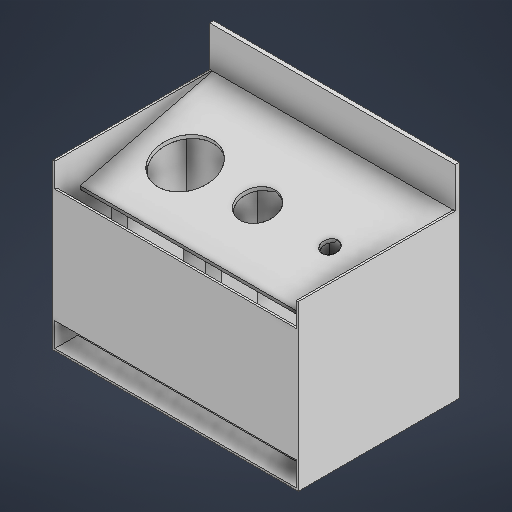
# Autodesk Inventor part: collectingbox
Saved by Autodesk Inventor 2026.2 (Build 302298000, 298)
## iProperties
Created: 2026-03-08
Part Number: collectingbox
Material: Generic
Document SubType Name: Modeling
Designer: danda
Density: 1 g/cm^3
Appearance: Default
Author: danda
Autodesk Inventor part; units mm, degrees
ref_plane "YZ Plane" through (0, 0, 0) normal (1, 0, 0) x (0, 1, 0)
ref_plane "XZ Plane" through (0, 0, 0) normal (0, 1, 0) x (-1, 0, 0)
ref_plane "XY Plane" through (0, 0, 0) normal (0, 0, 1) x (1, 0, 0)
sketch "Sketch1" plane through (0, 0, 0) normal (0, 0, 1) x (1, 0, 0)
  line L0 (-300, 0) -> (-300, 400)
  line L1 (-300, 0) -> (300, 0)
  line L2 (300, 0) -> (300, 400)
  line L3 (-305, 403.1883) -> (-305, -5)
  line L4 (-305, -5) -> (305, -5)
  line L5 (305, -5) -> (305, 403.1883)
  line L6 (-305, 403.1883) -> (305, 403.1883)
  line L7 (-305, 60) -> (300, 60)
  line L8 (-305, 303.1883) -> (305, 303.1883)
  point P0 (0, 0)
  point P1 (-300, 60)
  point P2 (300, 303.1883)
  point P3 (-300, 303.1883)
  dimension "d0" = 400
  dimension "d1" = 600
  dimension "d2" = 5
  dimension "d3" = 60
  dimension "d4" = 100
  dimension "d5" = 300
  constraints: 18 end point, 4 perpendicular, 4 point on line, 2 horizontal, 1 vertical, 2 other
  measures "d0" distance of L0.start L0.end
  measures "d1" distance of L0.start L1.end
  measures "d2" distance between parallel lines of L0 L3
  measures "d3" distance between parallel lines of L1 L7
  measures "d4" distance between parallel lines of L6 L8
  measures "d5" distance of L1.end point (0, 0)
extrude "Extrusion1" add sketch "Sketch1" along normal blind 400
extrude "Extrusion2" cut sketch "Sketch1" along normal blind 400 contours L0 L7 L2 L1
extrude "Extrusion3" add sketch "Sketch1" along normal blind 5 contours L0 L7 L2 L1
sketch "Sketch2" plane through (305, -5, 0) normal (1, 0, 0) x (0, 0, -1)
  line L0 (0, 0) -> (0, 408.1883) projected
  line L1 (0, 408.1883) -> (-400, 308.1883)
  line L2 (-400, 408.1883) -> (-400, 0) projected
  line L3 (-400, 308.1883) -> (-400, 408.1883)
  line L4 (0, 408.1883) -> (-400, 408.1883) projected
  line L5 (0, 408.1883) -> (-400, 408.1883)
  line L6 (-400, 408.1883) -> (0, 408.1883)
  line L7 (-400, 0) -> (-5, 34.558)
  line L8 (-5, 65) -> (-5, 5) projected
  line L9 (-400, 0) -> (-3.4912, 0) construction
  line L10 (-5, 34.558) -> (-5, 0)
  line L11 (0, 0) -> (-400, 0) projected
  line L12 (-5, 0) -> (-400, 0)
  line L13 (-400, 408.1883) -> (-395, 408.1883)
  line L14 (0, 408.1883) -> (-400, 408.1883) projected
  line L15 (-395, 408.1883) -> (-395, 309.4383)
  line L16 (-400, 308.1883) -> (-400, 408.1883)
  line L17 (-400, 308.1883) -> (-400, 348.1883)
  line L18 (-400, 348.1883) -> (-395, 348.1883)
  point P0 (0, 5)
  point P1 (-5, 5)
  dimension "d12" = 100
  dimension "d23" = 5
  dimension "d24" = 85
  dimension "d27" = 5
  dimension "d28" = 40
  constraints: 26 end point, 7 point on line, 4 collinear, 2 perpendicular, 1 equal length, 1 horizontal
  measures "d12" distance of L2.start L1.end
  measures "d23" angle of L9 L7
  measures "d24" angle of L7 L10
  measures "d27" distance of L2.start L13.end
  measures "d28" distance of L1.end L17.end
extrude "Extrusion4" cut sketch "Sketch2" against normal blind 605 contours L1 L15 L4 | L1 L2 L18 L15 | L15 L18 L2 L4
extrude "Extrusion5" add sketch "Sketch2" against normal blind 5 contours L1 L15 L4 | L1 L2 L18 L15 | L15 L18 L2 L4
extrude "Extrusion6" add sketch "Sketch2" against normal blind 5 contours L1 L15 L4 | L1 L2 L18 L15 | L15 L18 L2 L4
extrude "Extrusion7" cut sketch "Sketch1" along normal blind 395 contours L0 L8 L2 L7
extrude "Extrusion8" add sketch "Sketch1" along normal blind 5 contours L0 L8 L2 L7
extrude "Extrusion9" add sketch "Sketch2" against normal through all contours L11 L7 L8 L10
extrude "Extrusion10" add sketch "Sketch2" against normal through all contours L1 L2 L18 L15
sketch "Sketch3" plane through (-300, 403.1883, 0) normal (0, 0.9701425, 0.2425356) x (1, 0, 0)
  line L0 (600, -397.7584) -> (0, -397.7584) projected
  line L1 (600, -397.7584) -> (600, -347.7584)
  line L2 (600, -407.1567) -> (600, 0) projected
  arc A0 (214.6722, -335.3775) -> (214.6722, -335.3775) centre (157.4198, -2117.2252) ccw
  line L3 (600, -347.7584) -> (0, -347.7584)
  line L4 (0, -388.057) -> (0, 0) projected
  line L5 (0, -347.7584) -> (0, -397.7584)
  line L6 (0, -397.7584) -> (600, -397.7584)
  circle A1 centre (117.9242, -200) radius 70
  circle A2 centre (297.9242, -199.9892) radius 45
  circle A3 centre (477.9242, -200) radius 20
  line L7 (600, 0) -> (0, 0) projected
  point P0 (300, -97.7875)
  point P1 (300, 0)
  dimension "d31" = 50
  dimension "d32" = 140
  dimension "d33" = 90
  dimension "d34" = 40
  dimension "d35" = 200
  dimension "d36" = 200
  dimension "d37" = 200
  dimension "d38" = 180
  dimension "d39" = 180
  constraints: 8 end point, 4 centre point, 2 perpendicular, 2 point on circle, 2 point on line, 1 horizontal, 1 midpoint
  measures "d31" distance of L0.start L1.end
  measures "d32" diameter of A1
  measures "d33" diameter of A2
  measures "d34" diameter of A3
  measures "d35" distance from line of L7 A1.centre
  measures "d36" distance of point (300, 0) A2.centre
  measures "d37" distance from line of L7 A3.centre
  measures "d38" distance of A2.centre A1.centre
  measures "d39" distance of A3.centre A2.centre
extrude "Extrusion11" cut sketch "Sketch3" against normal blind 90 contours L0 L5 L4 L3 A0 L1 | A0 L3 L1 | A1 | A2 | A3
sketch "Sketch4" plane through (305, -5, 400) normal (1, 0, 0) x (0, 0, -1)
  line L0 (0, 408.1883) -> (400, 408.1883) projected
  line L1 (400, 408.1883) -> (62.6248, 323.8445) projected
  line L2 (400, 408.1883) -> (62.6248, 323.8445)
  line L3 (62.6248, 323.8445) -> (65.0501, 314.1431)
  line L4 (65.0501, 314.1431) -> (402.4254, 398.4869)
  line L5 (402.4254, 398.4869) -> (400, 408.1883)
  line L6 (395, 308.1883) -> (66.5388, 308.1883) projected
  line L7 (66.5388, 308.1883) -> (395, 308.1883)
  line L8 (395, 308.1883) -> (395, 396.6306)
  line L9 (65.0501, 314.1431) -> (66.5388, 308.1883)
  point P0 (400, 5)
  dimension "d42" = 10
  constraints: 14 end point, 3 equal length, 3 perpendicular, 1 point on line
  measures "d42" distance of L1.end L3.end
extrude "Extrusion12" cut sketch "Sketch4" against normal blind 605 contours L4 L8 L6 L9
extrude "Extrusion13" add sketch "Sketch4" against normal blind 5 contours L4 L8 L6 L9
sketch "Sketch5" plane through (-300, 304.4383, 395) normal (0, 0.9701425, 0.2425356) x (1, 0, 0)
  line L0 (0, 9.3983) -> (0, -0.3032) projected
  line L1 (0, -0.3032) -> (0, 9.3983)
  line L2 (600, 0) -> (600, 9.3983) projected
  line L3 (0, 9.3983) -> (600, 9.3983)
  line L4 (600, 9.3983) -> (600, 0)
  line L5 (600, 0) -> (0, -0.3032)
  line L6 (0, -0.3032) -> (600, 0)
  point P0 (300, 309.3691)
  constraints: 10 end point, 3 collinear, 1 perpendicular
extrude "Extrusion14" cut sketch "Sketch5" against normal blind 5
sketch "Sketch6" plane through (305, -5, 400) normal (1, 0, 0) x (0, 0, -1)
  line L0 (400, 0) -> (400, 408.1883) projected
  line L1 (400, 408.1883) -> (400, 508.1883)
  line L2 (400, 508.1883) -> (390, 508.1883)
  line L3 (390, 508.1883) -> (390, 408.1883)
  line L4 (0, 408.1883) -> (400, 408.1883) projected
  line L5 (390, 408.1883) -> (400, 408.1883)
  point P0 (400, 5)
  dimension "d49" = 100
  dimension "d50" = 10
  constraints: 8 end point, 2 perpendicular, 1 horizontal, 1 vertical
  measures "d49" distance of L0.end L1.end
  measures "d50" distance of L1.end L2.end
extrude "Extrusion15" add sketch "Sketch6" against normal blind 610
sketch "Sketch7" plane through (0, 0, 0) normal (0, 1, 0) x (-1, 0, 0)
  line L0 (252.0758, 120.8884) -> (112.0758, 120.8884)
  line L1 (112.0758, 120.8884) -> (112.0758, 267.1686)
  line L2 (252.0758, 267.1686) -> (252.0758, 120.8884)
  ellipse E0 centre (182.0758, 194.0285) end of major axis (112.0758, 194.0285) minor radius 67.91 projected
  line L3 (252.0758, 120.8884) -> (112.0758, 267.1686) construction
  line L4 (112.0758, 120.8884) -> (252.0758, 267.1686) construction
  line L5 (47.0758, 149.018) -> (-42.9242, 149.018)
  line L6 (-42.9242, 149.018) -> (-42.9242, 239.018)
  line L7 (47.0758, 239.018) -> (47.0758, 149.018)
  ellipse E1 centre (2.0758, 194.018) end of major axis (-42.9242, 194.018) minor radius 43.6564 projected
  line L8 (47.0758, 149.018) -> (-42.9242, 239.018) construction
  line L9 (-42.9242, 149.018) -> (47.0758, 239.018) construction
  line L10 (-157.9242, 174.0285) -> (-197.9242, 174.0285)
  line L11 (-197.9242, 174.0285) -> (-197.9242, 214.0285)
  line L12 (-157.9242, 214.0285) -> (-157.9242, 174.0285)
  ellipse E2 centre (-177.9242, 194.0285) end of major axis (-197.9242, 194.0285) minor radius 19.4029 projected
  line L13 (-157.9242, 174.0285) -> (-197.9242, 214.0285) construction
  line L14 (-197.9242, 174.0285) -> (-157.9242, 214.0285) construction
  line L15 (-217.9242, 154.0285) -> (-137.9242, 154.0285)
  line L16 (-137.9242, 154.0285) -> (-137.9242, 234.0285)
  line L17 (-217.9242, 234.0285) -> (-217.9242, 154.0285)
  line L18 (-62.9242, 129.018) -> (67.0758, 129.018)
  line L19 (67.0758, 129.018) -> (67.0758, 259.018)
  line L20 (-62.9242, 259.018) -> (-62.9242, 129.018)
  line L21 (92.5216, 100.8884) -> (272.0758, 100.8884)
  line L22 (272.0758, 100.8884) -> (272.0758, 286.31)
  line L23 (92.5216, 287.6) -> (92.5216, 100.8884)
  line L24 (272.0758, 286.31) -> (252.0758, 286.31)
  line L25 (112.0758, 287.6) -> (92.5216, 287.6)
  line L26 (67.0758, 259.018) -> (47.0758, 259.018)
  line L27 (-42.9242, 259.018) -> (-62.9242, 259.018)
  line L28 (-137.9242, 234.0285) -> (-157.9242, 234.0285)
  line L29 (-197.9242, 234.0285) -> (-217.9242, 234.0285)
  line L30 (92.5216, 287.6) -> (112.0758, 267.1686)
  line L31 (272.0758, 286.31) -> (252.0758, 267.1686)
  line L32 (67.0758, 259.018) -> (47.0758, 239.018)
  line L33 (-62.9242, 259.018) -> (-42.9242, 239.018)
  line L34 (-137.9242, 234.0285) -> (-157.9242, 214.0285)
  line L35 (-197.9242, 214.0285) -> (-217.9242, 234.0285)
  point P0 (0, 0)
  dimension "d55" = 20
  dimension "d56" = 20
  dimension "d57" = 20
  constraints: 72 end point, 12 parallel, 9 perpendicular, 6 midpoint, 6 point on line, 3 horizontal, 1 collinear, 6 other
  measures "d55" distance between parallel lines of L10 L15
  measures "d56" distance between parallel lines of L5 L18
  measures "d57" distance between parallel lines of L0 L21
extrude "Extrusion16" add sketch "Sketch7" along normal blind 370 contours L2 L31 L22 L21 L23 L30 L1 L0 | L7 L32 L19 L18 L20 L33 L6 L5 | L12 L34 L16 L15 L17 L35 L11 L10
ref_plane "Work Plane1" through (-300, 318.8445, 337.3752) normal (0, 0.9701425, 0.2425356) x (1, 0, 0)
sketch "Sketch8" plane through (217.9242, 344.6812, 234.0285) normal (1, 0, 0) x (0, 0, -1)
  line L0 (224.0285, 58.5071) -> (-165.9715, 58.5071) projected
  line L1 (224.0285, 58.5071) -> (-160.9715, -20.8679)
  line L2 (-160.9715, -40.2429) -> (-160.9715, -1.4929) projected
  line L3 (-103.3467, -25.8367) -> (234.0285, 58.5071) projected
  line L4 (229.0285, 46.9494) -> (-100.9214, -35.5381) projected
  line L5 (-103.3467, -25.8367) -> (-100.9214, -35.5381)
  line L6 (-100.9214, -35.5381) -> (229.0285, 46.9494)
  line L7 (229.0285, 46.9494) -> (224.0285, 58.5071)
  line L8 (-100.9214, -35.5381) -> (-100.9214, 58.5071)
  line L9 (-100.9214, 58.5071) -> (224.0285, 58.5071)
  line L10 (229.0285, 46.9494) -> (229.0285, -315.1232) projected
  line L11 (229.0285, 46.9494) -> (-100.9214, -35.5381)
  point P0 (234.0285, -344.6812)
  point P1 (-100.9214, -25.2303)
  point P2 (225.0045, 56.2511)
  constraints: 14 end point, 2 collinear, 2 perpendicular, 1 midpoint, 1 vertical
extrude "Extrusion17" cut sketch "Sketch8" against normal blind 500 contours L1 L8 L0 | L7 L3 L8 L1
equation "\"d36\" = d35"
equation "\"d37\" = d35"
equation "\"d39\" = d38"
body "Solid1"
